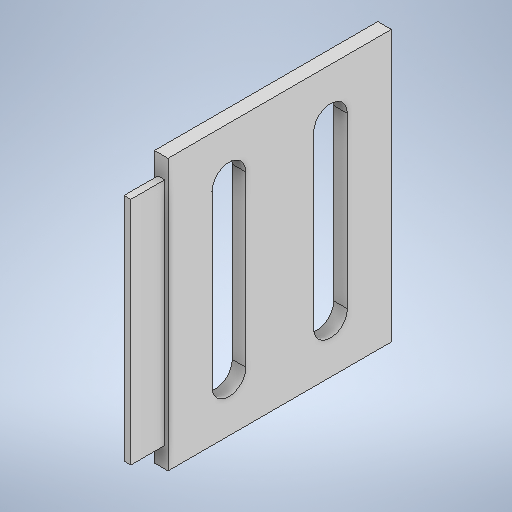
# Autodesk Inventor part: TSU_FM_Side_Wall
Saved by Autodesk Inventor 2025.2 (Build 292293000, 293)
## iProperties
Created: 2025-01-07
Part Number: TSU_FM_Side_Wall
Material: Generic
Document SubType Name: Modeling
Designer: Matt Tidd
Density: 1 g/cm^3
Appearance: Default
Author: Matt Tidd
Autodesk Inventor part; units mm, degrees
ref_plane "YZ Plane" through (0, 0, 0) normal (1, 0, 0) x (0, 1, 0)
ref_plane "XZ Plane" through (0, 0, 0) normal (0, 1, 0) x (-1, 0, 0)
ref_plane "XY Plane" through (0, 0, 0) normal (0, 0, 1) x (1, 0, 0)
sketch "Sketch1" plane through (0, 0, 0) normal (0, 1, 0) x (-1, 0, 0)
  line L0 (0, 0) -> (10, 0)
  line L1 (10, 0) -> (10, -165)
  line L2 (10, -165) -> (0, -165)
  line L3 (0, -165) -> (0, 0)
  dimension "d0" = 10
  dimension "d1" = 165
  constraints: 8 end point, 2 parallel, 1 horizontal, 1 perpendicular
  measures "d0" distance of L1.end L2.end
  measures "d1" distance of L0.end L1.end
extrude "Extrusion1" add sketch "Sketch1" along normal blind 200
sketch "Sketch2" plane through (-10, 0, 0) normal (0, 0, 1) x (1, 0, 0)
  line L0 (2.5, 15) -> (7.5, 15)
  line L1 (7.5, 15) -> (7.5, 185)
  line L2 (7.5, 185) -> (2.5, 185)
  line L3 (2.5, 185) -> (2.5, 15)
  point P0 (10, 0)
  dimension "d4" = 5
  dimension "d5" = 170
  constraints: 8 end point, 2 parallel, 1 horizontal, 1 perpendicular
  measures "d4" distance of L2.end L1.end
  measures "d5" distance of L1.end L0.end
extrude "Extrusion2" add sketch "Sketch2" along normal blind 25
sketch "Sketch3" plane through (0, 0, -165) normal (0, 0, -1) x (-1, 0, 0)
  line L0 (2.5, 15) -> (7.5, 15)
  line L1 (7.5, 15) -> (7.5, 185)
  line L2 (7.5, 185) -> (2.5, 185)
  line L3 (2.5, 185) -> (2.5, 15)
  point P0 (0, 0)
  dimension "d8" = 5
  dimension "d9" = 170
  constraints: 8 end point, 2 parallel, 1 horizontal, 1 perpendicular
  measures "d8" distance of L2.end L1.end
  measures "d9" distance of L1.end L0.end
extrude "Extrusion3" cut sketch "Sketch3" against normal blind 25
sketch "Sketch4" plane through (-10, 0, -165) normal (-1, 0, 0) x (0, 0, 1)
  line L0 (0, 200) -> (165, 200) construction
  line L1 (82.5, 200) -> (82.5, 0) construction
  line L2 (0, 0) -> (165, 0) construction
  line L3 (107.5, 175) -> (132.5, 175)
  line L4 (132.5, 175) -> (132.5, 25)
  line L5 (132.5, 25) -> (107.5, 25)
  line L6 (107.5, 25) -> (107.5, 175)
  line L7 (57.5, 175) -> (32.5, 175)
  line L8 (32.5, 175) -> (32.5, 25)
  line L9 (32.5, 25) -> (57.5, 25)
  line L10 (57.5, 25) -> (57.5, 175)
  dimension "d12" = 25
  dimension "d13" = 150
  dimension "d14" = 25
  dimension "d15" = 150
  constraints: 18 end point, 4 parallel, 2 horizontal, 2 midpoint, 2 perpendicular, 1 point on line
  measures "d12" distance of L4.end L5.end
  measures "d13" distance of L3.end L4.end
  measures "d14" distance of L9.end L8.end
  measures "d15" distance of L8.end L7.end
extrude "Extrusion4" cut sketch "Sketch4" against normal blind 10
fillet "Fillet1" radius 12.5 8 edges at (-5, 175, -107.5) (-5, 175, -32.5) (-5, 175, -57.5) (-5, 175, -132.5) (-5, 25, -132.5) (-5, 25, -107.5) (-5, 25, -57.5) (-5, 25, -32.5)
body "Solid1"
